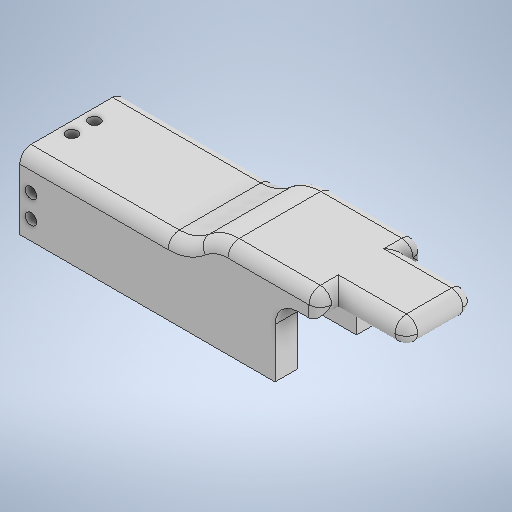
# Autodesk Inventor part: pulley_case_part_2
Saved by Autodesk Inventor 2025 (Build 290162000, 162)
## iProperties
Created: 2025-01-31
Part Number: pulley_case_part_2
Material: Generic
Document SubType Name: Modeling
Designer: danielrachi
Density: 1 g/cm^3
Appearance: Default
Author: danielrachi
Autodesk Inventor part; units mm, degrees
ref_plane "YZ Plane" through (0, 0, 0) normal (1, 0, 0) x (0, 1, 0)
ref_plane "XZ Plane" through (0, 0, 0) normal (0, 1, 0) x (-1, 0, 0)
ref_plane "XY Plane" through (0, 0, 0) normal (0, 0, 1) x (1, 0, 0)
sketch "Sketch1" plane through (0, 0, 0) normal (1, 0, 0) x (0, 1, 0)
  line L0 (-16, 23) -> (16, 23)
  line L1 (16, 23) -> (16, -23)
  line L2 (16, -23) -> (-16, -23)
  line L3 (-16, -23) -> (-16, 23)
  line L4 (-16, 23) -> (16, -23) construction
  line L5 (16, 23) -> (-16, -23) construction
  line L6 (-16, -18) -> (-16, 18)
  line L7 (-16, 13) -> (6, 13)
  line L8 (6, 13) -> (6, -13)
  line L9 (6, -13) -> (-16, -13)
  line L10 (-16, -13) -> (-16, 13)
  point P0 (0, 0)
  point P1 (-16, -13)
  dimension "d0" = 32
  dimension "d1" = 46
  dimension "d5" = 10
  dimension "d6" = 10
  dimension "d7" = 10
  constraints: 22 end point, 4 parallel, 2 horizontal, 2 midpoint, 2 perpendicular, 2 point on line
  measures "d0" distance of L1.end L2.end
  measures "d1" distance of L0.end L1.end
  measures "d5" distance between parallel lines of L0 L7
  measures "d6" distance between parallel lines of L9 L2
  measures "d7" distance between parallel lines of L8 L1
extrude "Extrusion1" add sketch "Sketch1" along normal blind 147.826 contours L0 L1 L2 L3 L9 L8 L7
sketch "Sketch2" plane through (0, 0, 0) normal (-1, 0, 0) x (0, 0, 1)
  line L0 (-13, -16) -> (-23, -16) projected
  line L1 (-18.25, -16) -> (18.25, -16)
  line L2 (18.25, -16) -> (18.25, 11.5)
  line L3 (18.25, 11.5) -> (-18.25, 11.5)
  line L4 (-18.25, 11.5) -> (-18.25, -16)
  line L5 (-23, -16) -> (-23, 16) projected
  line L6 (-23, 16) -> (23, 16) projected
  line L7 (23, 16) -> (23, -16) projected
  line L8 (-23, -16) -> (23, -16)
  line L9 (23, -16) -> (23, 16)
  line L10 (23, 16) -> (-23, 16)
  line L11 (-23, 16) -> (-23, -16)
  point P0 (0, 0)
  dimension "d10" = 4.75
  dimension "d11" = 4.5
  dimension "d12" = 4.75
  constraints: 16 end point, 4 parallel, 2 horizontal, 2 perpendicular, 1 point on line
  measures "d10" distance between parallel lines of L4 L5
  measures "d11" distance between parallel lines of L3 L6
  measures "d12" distance between parallel lines of L7 L2
extrude "Extrusion2" cut sketch "Sketch2" against normal blind 10 contours L0 L4 L3 L2 L1
sketch "Sketch3" plane through (0, 11.5, -18.25) normal (0, -1, 0) x (1, 0, 0)
  line L0 (0, 18.25) -> (10, 18.25)
  line L1 (10, 31.25) -> (10, 5.25) projected
  circle A0 centre (5, 23.25) radius 2.5
  circle A1 centre (5, 13.25) radius 2.5
  point P0 (5, 18.25)
  dimension "d15" = 5
  dimension "d16" = 5
  constraints: 2 centre point, 2 end point, 2 midpoint, 1 symmetric about line, 1 vertical alignment, 1 other
  measures "d15" diameter of A0
  measures "d16" distance from line of A0.centre L0
sketch "Sketch4" plane through (0, -16, -18.25) normal (0, 0, 1) x (1, 0, 0)
  line L0 (10, 27.5) -> (10, 0) projected
  line L1 (10, 22) -> (10, 0) projected
  line L2 (0, 0) -> (0, 27.5) projected
  circle A0 centre (5, 18.5) radius 2.5
  circle A1 centre (5, 8.5) radius 2.5
  line L3 (10, 0) -> (10, 27.5) projected
  line L4 (10, 13.75) -> (0, 13.75)
  point P0 (0, 16)
  point P1 (5, 13.75)
  dimension "d17" = 5
  dimension "d23" = 4.75
  dimension "d24" = 5.25
  dimension "d25" = 5
  constraints: 3 midpoint, 2 centre point, 2 end point, 2 vertical alignment
  measures "d17" diameter of A0
  measures "d23" distance from line of L4 A0.centre
  measures "d24" distance from line of A1.centre L4
  measures "d25" diameter of A1
extrude "Extrusion3" cut sketch "Sketch4" along normal through all both and the other way through all
extrude "Extrusion4" cut sketch "Sketch3" against normal blind 10
sketch "Sketch7" plane through (147.826, 0, 0) normal (1, 0, 0) x (0, 0, -1)
  line L0 (-15, 16) -> (-15, -16) projected
  line L1 (15, -16) -> (15, 16) projected
  line L2 (-15, 16) -> (15, 16)
  line L3 (15, 16) -> (15, 6)
  line L4 (15, 6) -> (-15, 6)
  line L5 (-15, 6) -> (-15, 16)
  line L6 (-13, 6) -> (13, 6) projected
  point P0 (0, 0)
  constraints: 8 end point, 2 collinear, 2 parallel, 1 horizontal, 1 perpendicular, 1 point on line
extrude "Extrusion7" add sketch "Sketch7" along normal blind 15
sketch "Sketch9" plane through (0, 16, 23) normal (0, 1, 0) x (1, 0, 0)
  line L0 (162.826, 38) -> (162.826, 8) projected
  line L1 (162.826, 38) -> (132.826, 38)
  line L2 (132.826, 38) -> (132.826, 8)
  line L3 (132.826, 8) -> (162.826, 8)
  line L4 (162.826, 8) -> (162.826, 38)
  line L5 (147.826, 8) -> (162.826, 8) projected
  point P0 (0, 23)
  dimension "d43" = 30
  constraints: 8 end point, 2 parallel, 1 collinear, 1 horizontal, 1 perpendicular
  measures "d43" distance of L3.end L2.end
extrude "Extrusion8" add sketch "Sketch9" along normal blind 10
sketch "Sketch10" plane through (10, 6, -13) normal (0, -1, 0) x (1, 0, 0)
  line L0 (152.826, 28) -> (152.826, -2) projected
  line L1 (152.826, 28) -> (122.826, 28)
  line L2 (122.826, 28) -> (122.826, -2)
  line L3 (122.826, -2) -> (152.826, -2)
  line L4 (152.826, -2) -> (152.826, 28)
  point P0 (-10, 13)
  dimension "d46" = 30
  constraints: 8 end point, 2 parallel, 1 horizontal, 1 perpendicular
  measures "d46" distance of L3.end L2.end
extrude "Extrusion9" cut sketch "Sketch10" along normal blind 30 and the other way blind 10
sketch "Sketch11" plane through (10, 16, -13) normal (0, -1, 0) x (1, 0, 0)
  circle A0 centre (137.826, 13) radius 10.125
  line L0 (152.826, 28) -> (152.826, -2) projected
  point P0 (-10, 13)
  point P1 (152.826, 13)
  point P2 (137.826, -2)
  dimension "d51" = 20.25
  constraints: 1 centre point, 1 horizontal alignment, 1 midpoint, 1 vertical alignment
  measures "d51" diameter of A0
extrude "Extrusion10" cut sketch "Sketch11" against normal blind 6
sketch "Sketch13" plane through (0, -16, 23) normal (0, 0, 1) x (1, 0, 0)
  line L0 (147.826, 0) -> (147.826, 32) projected
  line L1 (132.826, 32) -> (132.826, 42) projected
  line L2 (147.826, 0) -> (132.826, 0)
  line L3 (132.826, 0) -> (132.826, 32)
  line L4 (132.826, 32) -> (147.826, 32)
  line L5 (147.826, 32) -> (147.826, 0)
  point P0 (0, 16)
  constraints: 8 end point, 2 parallel, 1 horizontal, 1 perpendicular
extrude "Extrusion12" cut sketch "Sketch13" against normal through all
sketch "Sketch14" plane through (0, 16, 23) normal (0, 1, 0) x (1, 0, 0)
  line L0 (132.826, 0) -> (132.826, 8) projected
  line L1 (132.826, 0) -> (82.826, 0)
  line L2 (82.826, 0) -> (82.826, 46)
  line L3 (82.826, 46) -> (132.826, 46)
  line L4 (132.826, 46) -> (132.826, 0)
  line L5 (0, 46) -> (132.826, 46) projected
  point P0 (0, 23)
  dimension "d62" = 50
  constraints: 8 end point, 2 parallel, 1 collinear, 1 horizontal, 1 perpendicular
  measures "d62" distance of L2.end L3.end
extrude "Extrusion13" add sketch "Sketch14" along normal blind 10
sketch "Sketch15" plane through (0, -16, 23) normal (0, 0, 1) x (1, 0, 0)
  line L0 (0, 0) -> (132.826, 0) projected
  line L1 (132.826, 0) -> (112.826, 0)
  line L2 (112.826, 0) -> (112.826, 32)
  line L3 (112.826, 32) -> (132.826, 32)
  line L4 (132.826, 32) -> (132.826, 0)
  line L5 (0, 32) -> (82.826, 32) projected
  point P0 (0, 16)
  point P1 (112.826, 0)
  dimension "d65" = 20
  constraints: 8 end point, 2 parallel, 1 collinear, 1 horizontal, 1 perpendicular
  measures "d65" distance of L2.end L3.end
extrude "Extrusion14" cut sketch "Sketch15" against normal through all
fillet "Fillet1" radius 20 2 edges at (82.826, 26, 0) (82.826, 16, 0)
fillet "Fillet4" radius 10 1 edges at (112.826, 16, 0)
fillet "Fillet5" radius 5 4 edges at (112.3945, 26, 23) (32.7527, 16, 23) (112.3945, 26, -23) (32.7527, 16, -23)
fillet "Fillet6" radius 5 15 edges at (162.826, 21, 15) (162.826, 21, -15) (147.826, 26, 15) (162.826, 26, 0) (147.826, 26, -15) (132.826, 26, 16.5) (132.826, 18.5, 23) (132.826, 24.5355, 21.5355) (132.826, 24.5355, -21.5355) (132.826, 18.5, -23) (147.826, 16, 15) (132.826, 16, 19) (162.826, 16, 0) (147.826, 16, -15) (132.826, 16, -19)
sketch "Sketch18" plane through (0, -16, 18.25) normal (0, -1, 0) x (1, 0, 0)
  line L0 (10, -5.25) -> (102.826, -5.25)
  circle A0 centre (20, -0.25) radius 2.05
  line L1 (10, 0) -> (10, -5.25) projected
  line L2 (10, -5.25) -> (10, -31.25) projected
  line L3 (10, -18.25) -> (101.9239, -18.25)
  line L4 (101.9239, -5.25) -> (101.9239, -31.25) projected
  circle A1 centre (40, -0.25) radius 2.05
  circle A2 centre (60, -0.25) radius 2.05
  circle A3 centre (20, -36.25) radius 2.05
  circle A4 centre (40, -36.25) radius 2.05
  circle A5 centre (60, -36.25) radius 2.05
  point P0 (0, -18.25)
  dimension "d81" = 4.1
  dimension "d83" = 10
  dimension "d84" = 5
  dimension "d87" = 20
  constraints: 6 centre point, 4 end point, 3 symmetric about line, 2 horizontal, 2 midpoint, 7 other
  measures "d81" diameter of A0
  measures "d83" distance from line of A0.centre L1
  measures "d84" distance from line of A0.centre L0
  measures "d87" distance of A0.centre A1.centre
extrude "Extrusion17" cut sketch "Sketch18" against normal blind 5 contours A0 | A1 | A2 | A3 | A4 | A5
equation "\"d8\" = len"
equation "\"len_used_by_part1\" = 42.174"
equation "\"len\" = 147.826"
body "Solid1"
